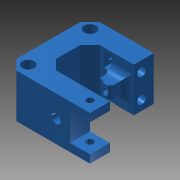
# Autodesk Inventor part: Infill3DBody
Saved by Autodesk Inventor 2015 SP1 (Build 190203100, 203)
## iProperties
Created: 2015-04-27
Part Number: Infill3DBody
Material: Generic
Document SubType Name: Modeling
Designer: Jack
Density: 1 g/cm^3
Appearance: Cyan
Author: Jack
Autodesk Inventor part; units mm, degrees
ref_plane "YZ Plane" through (0, 0, 0) normal (1, 0, 0) x (0, 1, 0)
ref_plane "XZ Plane" through (0, 0, 0) normal (0, 1, 0) x (-1, 0, 0)
ref_plane "XY Plane" through (0, 0, 0) normal (0, 0, 1) x (1, 0, 0)
sketch "Sketch1" plane through (0, 0, 0) normal (0, 0, 1) x (1, 0, 0)
  line L0 (42, 0) -> (0, 0)
  line L1 (0, 0) -> (0, 42)
  line L2 (0, 42) -> (42, 42)
  line L3 (42, 42) -> (42, 0)
  dimension "d3" = 42
  dimension "d4" = 42
  constraints: 8 end point, 2 parallel, 1 coincident, 1 horizontal, 1 perpendicular
  measures "d3" distance of L1.end L2.end
  measures "d4" distance of L0.end L1.end
extrude "Extrusion1" add sketch "Sketch1" along normal blind 22
sketch "Sketch2" plane through (0, 0, 22) normal (0, 0, 1) x (1, 0, 0)
  line L0 (0, 0) -> (42, 0) projected
  line L1 (0, 42) -> (0, 0) projected
  point P0 (5.5, 36.5)
  point P1 (5.5, 5.5)
  point P2 (36.5, 5.5)
  dimension "d9" = 31
  dimension "d10" = 31
  dimension "d11" = 5.5
  dimension "d12" = 5.5
  constraints: 1 horizontal alignment, 1 vertical alignment
  measures "d9" distance of point (5.5, 36.5) point (5.5, 5.5)
  measures "d10" distance of point (36.5, 5.5) point (5.5, 5.5)
  measures "d11" distance from line of L0 point (36.5, 5.5)
  measures "d12" distance from line of L1 point (5.5, 5.5)
hole "Hole1" at (5.5, 36.5, 22) at (5.5, 5.5, 22) direction (0, 0, -1) diameter 3.5 end through all counterbore diameter 6 counterbore depth 16
sketch "Sketch3" plane through (0, 0, 22) normal (0, 0, 1) x (1, 0, 0)
  line L0 (0, 0) -> (42, 0) projected
  line L1 (42, 42) -> (0, 42) projected
  line L2 (0, 42) -> (0, 0) projected
  line L3 (42, 42) -> (42, 0) projected
  line L4 (42, 32) -> (10, 32)
  line L5 (10, 32) -> (10, 10)
  line L6 (10, 10) -> (42, 10)
  dimension "d20" = 10
  dimension "d21" = 10
  dimension "d22" = 10
  constraints: 6 end point, 2 point on line, 1 horizontal, 1 perpendicular, 1 vertical
  measures "d20" distance between parallel lines of L0 L6
  measures "d21" distance between parallel lines of L2 L5
  measures "d22" distance between parallel lines of L1 L4
extrude "Extrusion2" cut sketch "Sketch3" against normal up to next contours L6 L5 L4 L3
sketch "Sketch4" plane through (42, 42, 22) normal (1, 0, 0) x (0, 0, -1)
  line L0 (0, -10) -> (22, -10) projected
  line L1 (22, 0) -> (22, -10) projected
  line L2 (22, 0) -> (0, 0) projected
  line L3 (0, -10) -> (0, 0) projected
extrude "Extrusion3" cut sketch "Sketch4" against normal blind 10
ref_plane "Work Plane1" through (24.5, 0, 0) normal (-1, 0, 0) x (0, 0, 1)
sketch "Sketch7" plane through (24.5, 0, 0) normal (-1, 0, 0) x (0, 0, 1)
  line L0 (0, 10) -> (22, 10) projected
  line L1 (14, 10) -> (14, 16.3)
  line L2 (14, 16.3) -> (8, 16.3)
  line L3 (8, 16.3) -> (8, 10)
  line L4 (0, 10) -> (0, 0) projected
  dimension "d45" = 6
  dimension "d46" = 8
  dimension "d47" = 6.3
  constraints: 6 end point, 2 perpendicular, 2 point on line, 1 vertical
  measures "d45" distance of L1.end L2.end
  measures "d46" distance between parallel lines of L4 L3
  measures "d47" distance of L1.start L1.end
extrude "Extrusion4" add sketch "Sketch7" along normal mid plane 6.5
ref_plane "Work Plane2" through (24.5, 0, 0) normal (-1, 0, 0) x (0, 0, 1)
sketch "Sketch8" plane through (24.5, 0, 0) normal (-1, 0, 0) x (0, 0, 1)
  line L0 (0, 32) -> (22, 32) projected
  line L1 (14, 32) -> (14, 25.7)
  line L2 (14, 25.7) -> (8, 25.7)
  line L3 (8, 25.7) -> (8, 32)
  line L4 (22, 32) -> (22, 42) projected
  point P0 (0, 0)
  dimension "d51" = 6
  dimension "d52" = 6.3
  dimension "d53" = 8
  constraints: 6 end point, 2 perpendicular, 2 point on line, 1 vertical
  measures "d51" distance of L1.end L2.end
  measures "d52" distance of L2.end L3.end
  measures "d53" distance between parallel lines of L4 L1
extrude "Extrusion5" add sketch "Sketch8" along normal mid plane 6.5
chamfer "Chamfer2" distance 1 angle 45 1 edges at (27.75, 16.3, 11)
sketch "Sketch14" plane through (21.25, 16.3, 14) normal (0, 0, 1) x (1, 0, 0)
  line L0 (0, 0) -> (6.5, 0) projected
  arc A0 (0, 0) -> (2.7877, 0.9675) centre (0, 4.5) ccw
  line L1 (5.5, 0) -> (6.5, -1) projected
  arc A1 (4.7877, 0.9675) -> (5.5, 0) centre (8.3284, 2.8284) ccw
  line L2 (2.7877, 0.9675) -> (4.7877, 0.9675)
  point P0 (-21.25, -16.3)
  dimension "d93" = 4
  dimension "d94" = 4.5
  dimension "d95" = 2
  constraints: 4 point on circle, 2 centre point, 2 end point, 2 tangent, 1 horizontal
  measures "d93" radius of A1
  measures "d94" radius of A0
  measures "d95" distance of L2.start L2.end
extrude "Extrusion9" add sketch "Sketch14" against normal up to surface (6 mm away)
sketch "Sketch15" plane through (21.25, 32, 14) normal (0, 0, 1) x (1, 0, 0)
  line L0 (6.5, -6.3) -> (0, -6.3) projected
  arc A0 (3.2619, -7.7) -> (0, -6.3) centre (0, -10.8) ccw
  line L1 (3.2619, -7.7) -> (5.2619, -7.7)
  arc A1 (6.5, -6.3) -> (5.2619, -7.7) centre (8.7944, -9.5765) ccw
  point P0 (-21.25, -32)
  dimension "d98" = 4.5
  dimension "d99" = 4
  dimension "d100" = 2
  dimension "d101" = 1.4
  constraints: 4 point on circle, 2 centre point, 2 end point, 1 horizontal, 1 tangent
  measures "d98" radius of A0
  measures "d99" radius of A1
  measures "d100" distance of L1.start L1.end
  measures "d101" distance between parallel lines of L0 L1
extrude "Extrusion10" add sketch "Sketch15" against normal up to surface (6 mm away)
sketch "Sketch5" plane through (0, 42, 22) normal (0, 1, 0) x (1, 0, 0)
  line L0 (0, 22) -> (32, 22) projected
  line L1 (0, 22) -> (0, 0) projected
  point P0 (25, 11)
  dimension "d27" = 11
  dimension "d29" = 25
  measures "d27" distance from line of L0 point (25, 11)
  measures "d29" distance from line of L1 point (25, 11)
hole "Hole2" at (25, 42, 11) direction (0, -1, 0) diameter 2 end through all
sketch "Sketch6" plane through (0, 0, 0) normal (0, -1, 0) x (1, 0, 0)
  circle A0 centre (25, 11) radius 1 projected
hole "Hole3" at (25, 0, 11) direction (0, 1, 0) diameter 4.5 depth 6 tip angle 90
sketch "Sketch10" plane through (0, 0, 0) normal (0, 0, -1) x (-1, 0, 0)
  line L0 (-10, 32) -> (-10, 10) projected
  line L1 (-10, 10) -> (-42, 10) projected
  circle A0 centre (-21, 21) radius 11.25
  dimension "d63" = 11
  dimension "d64" = 11
  dimension "d65" = 22.5
  constraints: 1 centre point, 1 coincident
  measures "d63" distance from line of L1 point (-21, 21)
  measures "d64" distance from line of L0 point (-21, 21)
  measures "d65" diameter of A0
extrude "Extrusion6" cut sketch "Sketch10" against normal blind 3 contours A0 L0 | L0 A0 L1 | L1 A0 picked at (-18.1333, 21.9679)
sketch "Sketch11" plane through (0, 0, 22) normal (0, 0, 1) x (1, 0, 0)
  circle A0 centre (5.5, 5.5) radius 3 projected
  point P0 (36.5, 5.5)
  dimension "d69" = 31
  constraints: 1 horizontal alignment
  measures "d69" distance of A0.centre point (36.5, 5.5)
hole "Hole5" at (36.5, 5.5, 22) direction (0, 0, -1) diameter 3.5 end through all
sketch "Sketch13" plane through (42, 0, 22) normal (1, 0, 0) x (0, 0, -1)
  line L0 (22, 10) -> (0, 10) projected
  line L1 (22, 0) -> (0, 0) projected
  line L2 (22, 10) -> (22, 0) projected
  line L3 (4, 10) -> (4, 0)
  line L4 (18, 0) -> (18, 10)
  dimension "d83" = 14
  dimension "d84" = 4
  constraints: 4 end point, 4 point on line, 2 perpendicular
  measures "d83" distance between parallel lines of L4 L3
  measures "d84" distance between parallel lines of L2 L4
extrude "Extrusion8" cut sketch "Sketch13" against normal blind 10 contours L4 L1 L3 L0
chamfer "Chamfer1" distance 5 angle 45 4 edges at (0, 42, 11) (0, 0, 11) (10, 10, 11) (10, 32, 11)
chamfer "Chamfer3" distance 1 angle 45 2 edges at (25.9677, 24.3, 10.7478) (24.7478, 24.3, 11.9677)
sketch "Sketch16" plane through (32, 42, 22) normal (1, 0, 0) x (0, 0, -1)
  line L0 (22, -10) -> (0, -10) projected
  line L1 (22, 0) -> (22, -10) projected
  point P0 (22, -42)
  point P1 (5, -6)
  point P2 (17, -6)
  dimension "d111" = 5
  dimension "d112" = 12
  dimension "d113" = 4
  constraints: 1 horizontal alignment
  measures "d111" distance from line of L1 point (17, -6)
  measures "d112" distance of point (5, -6) point (17, -6)
  measures "d113" distance from line of L0 point (5, -6)
hole "Hole6" at (32, 36, 17) at (32, 36, 5) direction (-1, 0, 0) diameter 4.5 depth 16
ref_plane "Work Plane3" through (17, 42, 22) normal (1, 0, 0) x (0, 0, -1)
fillet "Fillet1" radius 4 8 edges at (24.5, 10, 14) (27.75, 10, 11) (21.25, 10, 11) (24.5, 10, 8) (24.5, 32, 14) (27.75, 32, 11) (24.5, 32, 8) (21.25, 32, 11)
sketch "Sketch17" plane through (17, 42, 22) normal (1, 0, 0) x (0, 0, -1)
  circle A0 centre (5, -6) radius 2.25 projected
  circle A1 centre (17, -6) radius 2.25 projected
  line L0 (5, -10.2724) -> (1.3, -8.1362)
  line L1 (1.3, -8.1362) -> (1.3, -3.8638)
  line L2 (1.3, -3.8638) -> (5, -1.7276)
  line L3 (5, -1.7276) -> (8.7, -3.8638)
  line L4 (8.7, -3.8638) -> (8.7, -8.1362)
  line L5 (8.7, -8.1362) -> (5, -10.2724)
  line L6 (17, -10.2724) -> (13.3, -8.1362)
  line L7 (13.3, -8.1362) -> (13.3, -3.8638)
  line L8 (13.3, -3.8638) -> (17, -1.7276)
  line L9 (17, -1.7276) -> (20.7, -3.8638)
  line L10 (20.7, -3.8638) -> (20.7, -8.1362)
  line L11 (20.7, -8.1362) -> (17, -10.2724)
  line L12 (1.3, -8.1362) -> (1.3, -14)
  line L13 (1.3, -14) -> (8.7, -14)
  line L14 (8.7, -14) -> (8.7, -8.1362)
  line L15 (13.3, -8.1362) -> (13.3, -14)
  line L16 (13.3, -14) -> (20.7, -14)
  line L17 (20.7, -14) -> (20.7, -8.1362)
  point P0 (22, -42)
  dimension "d123" = 7.4
  dimension "d124" = 8
  constraints: 36 end point, 3 perpendicular, 3 vertical, 2 coincident, 2 parallel, 2 point on line, 1 horizontal alignment, 26 other
  measures "d123" distance between parallel lines of L1 L4
  measures "d124" distance from line of A1.centre L16
extrude "Extrusion11" cut sketch "Sketch17" along normal blind 3.8
body "Solid1"
